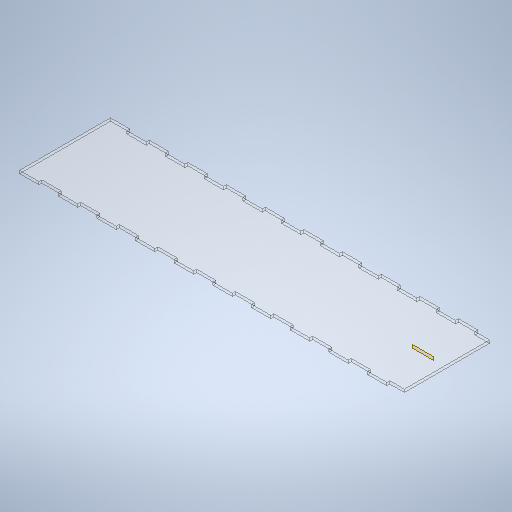
# Autodesk Inventor part: Part3 box.
Saved by Autodesk Inventor 2025.3 (Build 293356000, 356)
## iProperties
Created: 2026-04-07
Part Number: Part3 box.
Material: Acrylic
Document SubType Name: Modeling
Designer: logien
Density: 1.188 g/cm^3
Appearance: Transparent - Clear
Author: logien
Autodesk Inventor part; units mm, degrees
ref_plane "YZ Plane" through (0, 0, 0) normal (1, 0, 0) x (0, 1, 0)
ref_plane "XZ Plane" through (0, 0, 0) normal (0, 1, 0) x (-1, 0, 0)
ref_plane "XY Plane" through (0, 0, 0) normal (0, 0, 1) x (1, 0, 0)
sketch "Sketch1" plane through (0, 0, 0) normal (0, 1, 0) x (-1, 0, 0)
  line L0 (0, 0) -> (0, -88)
  line L1 (0, -88) -> (30, -88)
  line L2 (30, -88) -> (30, -91)
  line L3 (30, -91) -> (50, -91)
  line L4 (50, -91) -> (50, -88)
  line L5 (50, -88) -> (70, -88)
  line L6 (70, -88) -> (70, -91)
  line L7 (70, -91) -> (90, -91)
  line L8 (90, -91) -> (90, -88)
  line L9 (90, -88) -> (110, -88)
  line L10 (110, -88) -> (110, -91)
  line L11 (110, -91) -> (130, -91)
  line L12 (130, -91) -> (130, -88)
  line L13 (130, -88) -> (150, -88)
  line L14 (150, -88) -> (150, -91)
  line L15 (150, -91) -> (170, -91)
  line L16 (170, -91) -> (170, -88)
  line L17 (170, -88) -> (190, -88)
  line L18 (190, -88) -> (190, -91)
  line L19 (190, -91) -> (210, -91)
  line L20 (210, -91) -> (210, -88)
  line L21 (210, -88) -> (230, -88)
  line L22 (230, -88) -> (230, -91)
  line L23 (230, -91) -> (250, -91)
  line L24 (250, -91) -> (250, -88)
  line L25 (250, -88) -> (270, -88)
  line L26 (270, -88) -> (270, -91)
  line L27 (270, -91) -> (290, -91)
  line L28 (290, -91) -> (290, -88)
  line L29 (290, -88) -> (310, -88)
  line L30 (310, -88) -> (310, -91)
  line L31 (310, -91) -> (330, -91)
  line L32 (330, -91) -> (330, -88)
  line L33 (330, -88) -> (350, -88)
  line L34 (350, -88) -> (350, -91)
  line L35 (350, -91) -> (370, -91)
  line L36 (370, -91) -> (370, -88)
  line L37 (370, -88) -> (390, -88)
  line L38 (390, -88) -> (390, -91)
  line L39 (390, -91) -> (410, -91)
  line L40 (410, -91) -> (410, -88)
  line L41 (410, -88) -> (430, -88)
  line L42 (430, -88) -> (430, -91)
  line L43 (430, -91) -> (450, -91)
  line L44 (0, -44) -> (20, -44)
  line L45 (0, 0) -> (30, 0)
  line L46 (30, 0) -> (30, 3)
  line L47 (30, 3) -> (50, 3)
  line L48 (50, 3) -> (50, 0)
  line L49 (50, 0) -> (70, 0)
  line L50 (70, 0) -> (70, 3)
  line L51 (70, 3) -> (90, 3)
  line L52 (90, 3) -> (90, 0)
  line L53 (90, 0) -> (110, 0)
  line L54 (110, 0) -> (110, 3)
  line L55 (110, 3) -> (130, 3)
  line L56 (130, 3) -> (130, 0)
  line L57 (130, 0) -> (150, 0)
  line L58 (150, 0) -> (150, 3)
  line L59 (150, 3) -> (170, 3)
  line L60 (170, 3) -> (170, 0)
  line L61 (170, 0) -> (190, 0)
  line L62 (190, 0) -> (190, 3)
  line L63 (190, 3) -> (210, 3)
  line L64 (210, 3) -> (210, 0)
  line L65 (210, 0) -> (230, 0)
  line L66 (230, 0) -> (230, 3)
  line L67 (230, 3) -> (250, 3)
  line L68 (250, 3) -> (250, 0)
  line L69 (250, 0) -> (270, 0)
  line L70 (270, 0) -> (270, 3)
  line L71 (270, 3) -> (290, 3)
  line L72 (290, 3) -> (290, 0)
  line L73 (290, 0) -> (310, 0)
  line L74 (310, 0) -> (310, 3)
  line L75 (310, 3) -> (330, 3)
  line L76 (330, 3) -> (330, 0)
  line L77 (330, 0) -> (350, 0)
  line L78 (350, 0) -> (350, 3)
  line L79 (350, 3) -> (370, 3)
  line L80 (370, 3) -> (370, 0)
  line L81 (370, 0) -> (390, 0)
  line L82 (390, 0) -> (390, 3)
  line L83 (390, 3) -> (410, 3)
  line L84 (410, 3) -> (410, 0)
  line L85 (410, 0) -> (430, 0)
  line L86 (430, 0) -> (430, 3)
  line L87 (430, 3) -> (450, 3)
  line L88 (450, 3) -> (450, -91)
  dimension "d0" = 88
  dimension "d1" = 30
  dimension "d2" = 3
  dimension "d3" = 20
  dimension "d4" = 20
  dimension "d5" = 20
  dimension "d6" = 20
  dimension "d7" = 20
  dimension "d8" = 20
  dimension "d9" = 3
  dimension "d10" = 20
  dimension "d11" = 3
  dimension "d12" = 20
  dimension "d13" = 3
  dimension "d14" = 20
  dimension "d15" = 3
  dimension "d16" = 20
  dimension "d17" = 3
  dimension "d18" = 20
  dimension "d19" = 3
  dimension "d20" = 20
  dimension "d21" = 3
  dimension "d22" = 20
  dimension "d23" = 3
  dimension "d24" = 20
  dimension "d25" = 3
  dimension "d26" = 20
  dimension "d27" = 3
  dimension "d28" = 20
  dimension "d29" = 3
  dimension "d30" = 20
  dimension "d31" = 3
  dimension "d32" = 20
  dimension "d33" = 3
  dimension "d34" = 20
  dimension "d35" = 3
  dimension "d36" = 20
  dimension "d37" = 3
  dimension "d38" = 20
  dimension "d39" = 3
  dimension "d40" = 0
  dimension "d41" = 20
  constraints: 178 end point, 43 symmetric about line, 42 point on line, 18 perpendicular, 5 vertical, 4 horizontal, 1 midpoint, 1 parallel
  measures "d0" distance of L0.start L0.end
  measures "d1" distance of L0.end L1.end
  measures "d2" distance of L1.end L2.end
  measures "d3" distance of L2.end L3.end
  measures "d4" distance of L4.end L5.end
  measures "d5" distance of L6.end L7.end
  measures "d6" distance of L8.end L9.end
  measures "d7" distance of L10.end L11.end
  measures "d8" distance of L12.end L13.end
  measures "d9" distance of L13.end L14.end
  measures "d10" distance of L14.end L15.end
  measures "d11" distance of L15.end L16.end
  measures "d12" distance of L16.end L17.end
  measures "d13" distance of L17.end L18.end
  measures "d14" distance of L18.end L19.end
  measures "d15" distance of L19.end L20.end
  measures "d16" distance of L20.end L21.end
  measures "d17" distance of L21.end L22.end
  measures "d18" distance of L22.end L23.end
  measures "d19" distance of L23.end L24.end
  measures "d20" distance of L24.end L25.end
  measures "d21" distance of L25.end L26.end
  measures "d22" distance of L26.end L27.end
  measures "d23" distance of L27.end L28.end
  measures "d24" distance of L28.end L29.end
  measures "d25" distance of L29.end L30.end
  measures "d26" distance of L30.end L31.end
  measures "d27" distance of L31.end L32.end
  measures "d28" distance of L32.end L33.end
  measures "d29" distance of L33.end L34.end
  measures "d30" distance of L34.end L35.end
  measures "d31" distance of L35.end L36.end
  measures "d32" distance of L36.end L37.end
  measures "d33" distance of L37.end L38.end
  measures "d34" distance of L38.end L39.end
  measures "d35" distance of L39.end L40.end
  measures "d36" distance of L40.end L41.end
  measures "d37" distance of L41.end L42.end
  measures "d38" distance of L42.end L43.end
  measures "d39" distance between parallel lines of L9 L43
  measures "d40" distance between parallel lines of L7 L35
  measures "d41" distance of L44.start L44.end
extrude "Extrusion1" add sketch "Sketch1" along normal blind 3
sketch "Sketch2" plane through (0, 3, 0) normal (0, 1, 0) x (1, 0, 0)
  line L0 (0, 0) -> (0, 88) projected
  line L1 (0, 44) -> (-55, 44)
  line L2 (-55, 44) -> (-55, 97)
  line L3 (-55, 97) -> (0, 97)
  line L4 (0, 97) -> (0, -10)
  line L5 (0, -10) -> (-55, -10)
  line L6 (-55, -10) -> (-55, 44)
  dimension "d44" = 55
  dimension "d45" = 0
  constraints: 12 end point, 4 perpendicular, 1 collinear, 1 horizontal, 1 midpoint, 1 point on line
  measures "d44" distance of L1.start L1.end
  measures "d45" distance between parallel lines of L0 L4
extrude "Extrusion2" cut sketch "Sketch2" against normal blind 3
ref_plane "Work Plane1" through (-90, 0, -44) normal (0, 0, 1) x (1, 0, 0)
body "Solid1"
